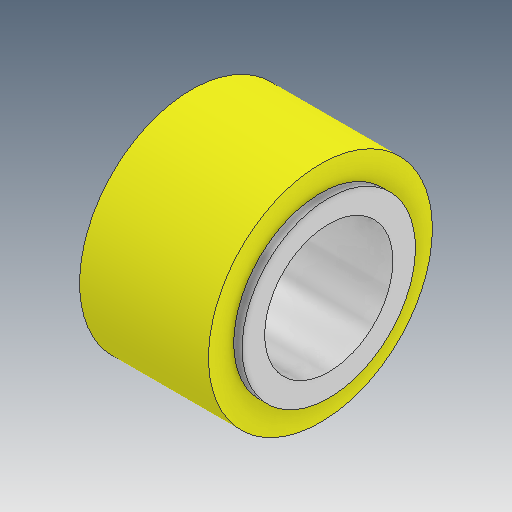
# Autodesk Inventor part: Roda
Saved by Autodesk Inventor 2026.1 (Build 301233020, 233B)
## iProperties
Created: 2025-11-09
Part Number: Roda
Material: Genérico
Document SubType Name: Modeling
Designer: Emmanuel Ribeiro
Density: 1 g/cm^3
Appearance: Padrão
Author: Emmanuel Ribeiro
Autodesk Inventor part; units mm, degrees
ref_plane "YZ Plane" through (0, 0, 0) normal (1, 0, 0) x (0, 1, 0)
ref_plane "XZ Plane" through (0, 0, 0) normal (0, 1, 0) x (-1, 0, 0)
sketch "Esboço1" plane through (0, 0, 0) normal (1, 0, 0) x (0, 1, 0)
  circle A0 centre (0, 0) radius 12.5
  circle A1 centre (0, 0) radius 2
  dimension "d0" = 25
  dimension "d1" = 4
  constraints: 2 centre point, 2 coincident
  measures "d0" diameter of A0
  measures "d1" diameter of A1
extrude "Extrusão1" add sketch "Esboço1" along normal blind 21
sketch "Esboço2" plane through (21, 0, 0) normal (1, 0, 0) x (0, 0, -1)
  circle A0 centre (0, 0) radius 9.25
  dimension "d4" = 18.5
  constraints: 1 centre point, 1 coincident
  measures "d4" diameter of A0
extrude "Extrusão2" cut sketch "Esboço2" against normal blind 14
ref_plane "Plano de trabalho1" through (19.8, 0, 0) normal (1, 0, 0) x (0, 0, -1)
sketch "Esboço3" plane through (19.8, 0, 0) normal (1, 0, 0) x (0, 0, -1)
  circle A0 centre (0, 0) radius 12.5 projected
  circle A1 centre (0, 0) radius 2 projected
  circle A2 centre (0, 0) radius 16.15
  dimension "d8" = 32.3
  constraints: 1 centre point, 1 coincident
  measures "d8" diameter of A2
extrude "Extrusão3" add sketch "Esboço3" against normal blind 18.6 separate body contours A2
